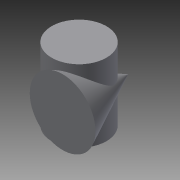
# Autodesk Inventor part: 第一次上机-模型1
Saved by Autodesk Inventor 2013 (Build 170138000, 138)
## iProperties
Created: 2016-11-06
Part Number: 第一次上机-模型1
Material: 常规
Document SubType Name: Modeling
Designer: Administrator
Density: 1 g/cm^3
Author: Administrator
Autodesk Inventor part; units mm, degrees
ref_plane "YZ Plane" through (0, 0, 0) normal (1, 0, 0) x (0, 1, 0)
ref_plane "XZ Plane" through (0, 0, 0) normal (0, 1, 0) x (-1, 0, 0)
ref_plane "XY Plane" through (0, 0, 0) normal (0, 0, 1) x (1, 0, 0)
sketch "草图2" plane through (0, 0, 0) normal (0, 1, 0) x (-1, 0, 0)
  circle A0 centre (0, 0) radius 30
  dimension "d0" = 60
  constraints: 1 centre point, 1 coincident
  measures "d0" diameter of A0
sketch "草图3" plane through (0, 0, 0) normal (1, 0, 0) x (0, 1, 0)
  point P0 (0, 0)
  point P1 (60, 0)
  dimension "d2" = 60
  measures "d2" distance of point (60, 0) point (0, 0)
loft "放样1" add profiles "草图2" section 1 point at (0, 60, 0)
sketch "草图4" plane through (0, 0, 0) normal (0, 0, 1) x (1, 0, 0)
  line L0 (30, 0) -> (-30, 0) projected
  line L1 (0, 60) -> (0, 0) construction
  circle A0 centre (-15, 30) radius 25
  point P0 (0, 60)
  dimension "d7" = 50
  dimension "d9" = 15
  dimension "d10" = 30
  constraints: 2 end point, 1 centre point, 1 perpendicular
  measures "d7" diameter of A0
  measures "d9" distance from line of L1 A0.centre
  measures "d10" distance from line of L0 A0.centre
extrude "拉伸1" add sketch "草图4" along normal mid plane 66
